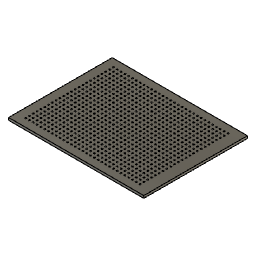
Universal90x70_200718_actualSize (Autodesk Fusion 360 design; units mm, degrees)
Autodesk Fusion 360 part; units mm, degrees
sketch "スケッチ1" plane through (0, 0, 0) normal (0, 0, 1) x (1, 0, 0)
  line L0 (0, 0) -> (90, 0)
  line L1 (90, 0) -> (90, 69)
  line L2 (90, 69) -> (0, 69)
  line L3 (0, 69) -> (0, 0)
  dimension "d1" = 90
  dimension "d2" = 69
  constraint horizontal L0
  constraint vertical L1
  constraint horizontal L2
  constraint vertical L3
  constraint coincident L0.start L3.end
  measures "d1" distance of L0.start L0.end
  measures "d2" distance of L0.start L2.end
extrude "押し出し1" add sketch "スケッチ1" along normal blind 1.6
sketch "スケッチ2" plane through (0, 0, 1.6) normal (0, 0, 1) x (-1, 0, 0)
  line L0 (0, -69) -> (0, 0)
  line L1 (0, 0) -> (-90, 0)
  line L2 (-90, 0) -> (-90, -69)
  line L3 (-90, -69) -> (0, -69)
  circle A0 centre (-6, -5.4) radius 0.5
  dimension "d5" = 1
  dimension "d6" = 5.4
  dimension "d7" = 6
  measures "d5" diameter of A0
  measures "d6" distance of L1 A0.centre
  measures "d7" distance of L0 A0.centre
extrude "押し出し2" cut sketch "スケッチ2" against normal blind 1.6 contours A0
pattern_linear "R パターン1" count 31 spacing 2.54 along (1, 0, 0) count 24 spacing 2.54 along (0, 1, 0) of "押し出し2"
